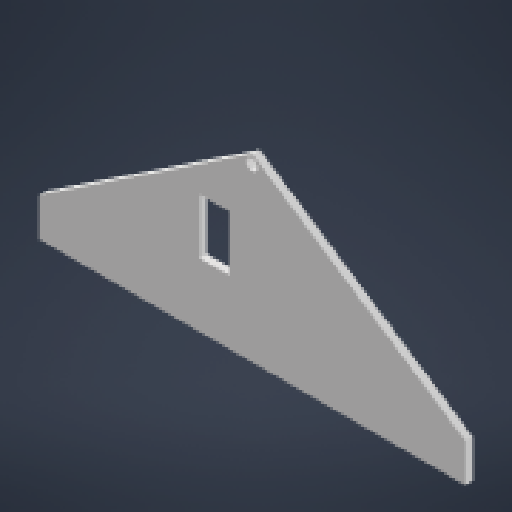
# Autodesk Inventor part: Pieza8
Saved by Autodesk Inventor 2026.1 (Build 301233020, 233B)
## iProperties
Created: 2026-05-06
Part Number: Pieza8
Material: Genérico
Document SubType Name: Modeling
Designer: OlmesTech
Density: 1 g/cm^3
Appearance: Valor por defecto
Author: OlmesTech
Autodesk Inventor part; units mm, degrees
ref_plane "YZ Plane" through (0, 0, 0) normal (1, 0, 0) x (0, 1, 0)
ref_plane "XZ Plane" through (0, 0, 0) normal (0, 1, 0) x (-1, 0, 0)
ref_plane "XY Plane" through (0, 0, 0) normal (0, 0, 1) x (1, 0, 0)
sketch "Boceto1" plane through (0, 0, 0) normal (0, 0, 1) x (1, 0, 0)
  arc A0 (-1.5, 113.1763) -> (1.5, 113.1763) centre (0, 113.1763) ccw
  line L0 (0, 113.1763) -> (0, 116.1763)
  line L1 (0, 117.735) -> (-0.0114, 117.7429)
  line L2 (0, 111.6763) -> (85, 55)
  line L3 (-2.22, 113.8018) -> (0.2156, 115.4258)
  line L4 (1.8799, 112.9298) -> (0.2156, 115.4258)
  line L5 (-0.5557, 111.3058) -> (1.8799, 112.9298)
  line L6 (1.8799, 112.9298) -> (0.2156, 115.4258)
  line L7 (-2.22, 113.8018) -> (0.2156, 115.4258)
  line L8 (-0.5557, 111.3058) -> (-2.22, 113.8018)
  line L9 (-2.22, 113.8018) -> (1.8799, 112.9298)
  line L10 (-0.5557, 111.3058) -> (0.2156, 115.4258)
  circle A1 centre (-0.17, 113.3658) radius 2.0958
  line L11 (85, 45) -> (85, 59.843)
  line L12 (-85, 45) -> (-85, 59.843)
  circle A2 centre (-0.17, 113.3658) radius 2.1904
  line L13 (-9, 92.5193) -> (-21, 92.5193)
  line L14 (-21, 92.5193) -> (-21, 70.5193)
  line L15 (-21, 70.5193) -> (-9, 70.5193)
  line L16 (-9, 70.5193) -> (-9, 92.5193)
  line L17 (-9, 92.5193) -> (-21, 70.5193)
  line L18 (-21, 92.5193) -> (-9, 70.5193)
  line L19 (85, 45) -> (-85, 45)
  line L20 (85, 49.7321) -> (85, 32.7679)
  line L21 (85, 49.7321) -> (85, 32.7679)
  line L22 (-85, 55) -> (0, 111.6763)
  line L23 (-85, 60.3554) -> (0, 117.0317)
  line L24 (0, 117.0317) -> (85, 60.3554)
  line L25 (85, 59.843) -> (85, 60.3554)
  line L26 (-85, 59.843) -> (-85, 60.3554)
  point P0 (0, 0)
  point P1 (96.4858, 46.8907)
  point P2 (-94.6783, 48.1668)
  point P3 (-94.6783, 45)
  point P4 (96.4858, 45)
  point P5 (-15, 81.5193)
  point P6 (0, 45)
  point P7 (-15, 81.5193)
extrude "Extrusión1" add sketch "Boceto1" along normal blind 3 contours L22 L12 L26 L23 L24 L25 L11 L2 A2 | A2 L2 L11 L19 L12 L22
